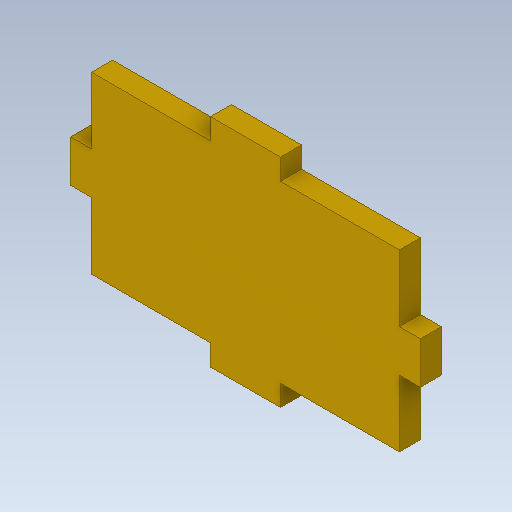
# Autodesk Inventor part: Part6
Saved by Autodesk Inventor 2020 (Build 240168000, 168)
## iProperties
Created: 2020-03-11
Part Number: Part6
Material: Generic
Document SubType Name: Modeling
Designer: tor16003
Density: 1 g/cm^3
Appearance: Gold
Author: tor16003
Autodesk Inventor part; units mm, degrees
ref_plane "YZ Plane" through (0, 0, 0) normal (1, 0, 0) x (0, 1, 0)
ref_plane "XZ Plane" through (0, 0, 0) normal (0, 1, 0) x (-1, 0, 0)
ref_plane "XY Plane" through (0, 0, 0) normal (0, 0, 1) x (1, 0, 0)
sketch "Sketch1" plane through (0, 0, 0) normal (0, 0, 1) x (1, 0, 0)
  line L0 (0, 9.5) -> (-3, 9.5)
  line L1 (-3, 9.5) -> (-3, 15.5)
  line L2 (-3, 15.5) -> (0, 15.5)
  line L3 (0, 15.5) -> (0, 25)
  line L4 (44, 25) -> (44, 15.5)
  line L5 (44, 15.5) -> (47, 15.5)
  line L6 (47, 15.5) -> (47, 9.5)
  line L7 (47, 9.5) -> (44, 9.5)
  line L8 (44, 9.5) -> (44, 0)
  line L9 (0, 0) -> (0, 9.5)
  line L10 (0, 25) -> (17, 25)
  line L11 (17, 25) -> (17, 28)
  line L12 (17, 28) -> (27, 28)
  line L13 (27, 28) -> (27, 25)
  line L14 (27, 25) -> (44, 25)
  line L15 (0, 0) -> (17, 0)
  line L16 (17, 0) -> (17, -3)
  line L17 (17, -3) -> (27, -3)
  line L18 (27, -3) -> (27, 0)
  line L19 (27, 0) -> (44, 0)
  dimension "d0" = 6
  dimension "d1" = 3
  dimension "d2" = 3
  dimension "d3" = 6
  dimension "d4" = 50
  dimension "d5" = 3
  dimension "d6" = 10
  dimension "d7" = 3
  dimension "d14" = 25
  constraints: 40 end point, 12 perpendicular, 7 point on line, 4 equal length, 3 horizontal, 2 coincident, 2 collinear, 1 vertical
  measures "d0" distance of L0.end L1.end
  measures "d1" distance of L1.end L2.end
  measures "d2" distance of L4.end L5.end
  measures "d3" distance of L5.end L6.end
  measures "d4" distance between parallel lines of L6 L1
  measures "d5" distance of L10.end L11.end
  measures "d6" distance between parallel lines of L13 L11
  measures "d7" distance of L15.end L16.end
  measures "d14" distance between parallel lines of L15 L10
extrude "Extrusion1" add sketch "Sketch1" along normal blind 3
body "Solid1"
